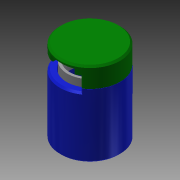
# Autodesk Inventor part: microscope_iphone_adapter
Saved by Autodesk Inventor 2014 (Build 180170000, 170)
## iProperties
Created: 2015-01-25
Part Number: microscope_iphone_adapter
Material: Generic
Document SubType Name: Modeling
Designer: caleb
Density: 1 g/cm^3
Appearance: Default
Author: caleb
Autodesk Inventor part; units mm, degrees
ref_plane "YZ Plane" through (0, 0, 0) normal (1, 0, 0) x (0, 1, 0)
ref_plane "XZ Plane" through (0, 0, 0) normal (0, 1, 0) x (-1, 0, 0)
ref_plane "XY Plane" through (0, 0, 0) normal (0, 0, 1) x (1, 0, 0)
sketch "Sketch1" plane through (0, 0, 0) normal (0, 0, 1) x (1, 0, 0)
  circle A0 centre (0, 0) radius 13.5
  dimension "d0" = 27
  constraints: 1 centre point, 1 coincident
  measures "d0" diameter of A0
extrude "Extrusion1" add sketch "Sketch1" against normal blind 25
ref_plane "Work Plane1" through (0, 0, 11) normal (0, 0, 1) x (1, 0, 0)
sketch "Sketch2" plane through (0, 0, 11) normal (0, 0, 1) x (1, 0, 0)
  circle A0 centre (0, 0) radius 13.9
  circle A1 centre (0, 0) radius 17.9
  circle A2 centre (0, 0) radius 13.5 construction
  dimension "d4" = 0.4
  dimension "d5" = 4
  constraints: 2 centre point, 2 coincident
  measures "d4" radial gap between concentric circles of A0 A2
  measures "d5" radial gap between concentric circles of A0 A1
extrude "Extrusion2" add sketch "Sketch2" against normal blind 36 separate body
sketch "Sketch3" plane through (0, 0, 11) normal (0, 0, 1) x (1, 0, 0)
  line L0 (9.28, 7.35) -> (-49.29, 7.35)
  line L1 (-49.29, 7.35) -> (-49.29, -116.48)
  line L2 (-49.29, -116.48) -> (9.28, -116.48)
  line L3 (9.28, -116.48) -> (9.28, 7.35)
  point P0 (0, 0)
  dimension "d8" = 58.57
  dimension "d9" = 123.83
  dimension "d10" = 9.28
  dimension "d11" = 7.35
  constraints: 8 end point, 2 parallel, 1 horizontal, 1 perpendicular
  measures "d8" distance of L1.end L2.end
  measures "d9" distance of L0.end L1.end
  measures "d10" distance from line of L3 point (0, 0)
  measures "d11" distance from line of L0 point (0, 0)
extrude "Extrusion3" add sketch "Sketch3" along normal blind 8.1 separate body
sketch "Sketch6" plane through (-49.29, 7.35, 11) normal (0, 1, 0) x (1, 0, 0)
  line L0 (58.57, 0) -> (0, 0) projected
  line L1 (0, 0) -> (0, -8.1) projected
  line L2 (58.57, -8.1) -> (0, -8.1) projected
  line L3 (58.57, 0) -> (58.57, -8.1) projected
  line L4 (38.77, -2.7) -> (49.27, -2.7)
  line L5 (49.27, -2.7) -> (49.27, -5.4)
  line L6 (49.27, -5.4) -> (38.77, -5.4)
  line L7 (38.77, -5.4) -> (38.77, -2.7)
  point P0 (49.29, 11)
  point P1 (49.27, -4.05)
  point P2 (58.57, -4.05)
  dimension "d20" = 10.5
  dimension "d21" = 2.7
  dimension "d22" = 9.3
  constraints: 8 end point, 2 midpoint, 2 parallel, 1 horizontal, 1 horizontal alignment, 1 perpendicular
  measures "d20" distance of L5.end L6.end
  measures "d21" distance of L4.end L5.end
  measures "d22" distance between parallel lines of L3 L5
extrude "Extrusion6" add sketch "Sketch6" along normal blind 1.08 contours L4 L5 L6 L7 bodies 3
fillet "Fillet1" radius 6 4 edges at (9.28, 7.35, 15.05) (-49.29, 7.35, 15.05) (9.28, -116.48, 15.05) (-49.29, -116.48, 15.05)
ref_plane "Work Plane2" through (0, 0, 20.9) normal (0, 0, 1) x (1, 0, 0)
sketch "Sketch4" plane through (0, 0, 11) normal (0, 0, 1) x (1, 0, 0)
  circle A0 centre (0, 0) radius 13.9 projected
  circle A1 centre (0, 0) radius 17.9 projected
extrude "Extrusion4" add sketch "Sketch4" along normal up to surface (9.9 mm away) bodies 2
sketch "Sketch5" plane through (0, 0, 20.9) normal (0, 0, 1) x (1, 0, 0)
  circle A0 centre (0, 0) radius 17.9 projected
extrude "Extrusion5" add sketch "Sketch5" along normal blind 4 bodies 2
combine bodies "Combine1" operation type subtract main body 2 bodies to subtract 3 keep tools yes
sketch "Sketch7" plane through (0, 0, 19.1) normal (0, 0, 1) x (1, 0, 0)
  arc A0 (-49.29, -110.48) -> (-43.29, -116.48) centre (-43.29, -110.48) ccw construction
  line L0 (-49.29, 1.35) -> (-49.29, -110.48) construction
  arc A1 (-43.29, 7.35) -> (-49.29, 1.35) centre (-43.29, 1.35) ccw construction
  line L1 (3.28, 7.35) -> (-43.29, 7.35) projected
  arc A2 (9.28, 1.35) -> (3.28, 7.35) centre (3.28, 1.35) ccw projected
  line L2 (9.28, -110.48) -> (9.28, 1.35) projected
  arc A3 (3.28, -116.48) -> (9.28, -110.48) centre (3.28, -110.48) ccw construction
  line L3 (-43.29, -116.48) -> (3.28, -116.48) construction
  line L4 (-0.02, 7.35) -> (-10.52, 7.35) construction
  line L5 (-0.02, 7.35) -> (-10.52, 7.35) construction
  line L6 (-0.02, 7.35) -> (-0.02, 8.43) construction
  line L7 (-10.52, 8.43) -> (-0.02, 8.43) construction
  line L8 (-10.52, 7.35) -> (-10.52, 8.43) construction
  circle A4 centre (0, 0) radius 13.9 construction
  circle A5 centre (0, 0) radius 17.9 construction
  arc A6 (9.28, -10.3485) -> (0.48, 13.8917) centre (0, 0) ccw
  line L9 (0.48, 13.8917) -> (0.48, 7.35)
  dimension "d25" = 0.5
  constraints: 4 point on circle, 2 concentric, 2 end point, 2 point on line, 1 centre point, 1 vertical
  measures "d25" distance between parallel lines of L9 L6
extrude "Extrusion7" add sketch "Sketch7" against normal blind 4 bodies 2
extrude "Extrusion8" add sketch "Sketch7" along normal up to next bodies 2
sketch "Sketch8" plane through (0, 0, 20.9) normal (0, 0, -1) x (-1, 0, 0)
  line L0 (-0.48, 13.8917) -> (-0.48, 7.35) projected
  line L1 (-0.48, 7.35) -> (-3.28, 7.35) projected
  arc A0 (-3.28, 7.35) -> (-9.28, 1.35) centre (-3.28, 1.35) ccw projected
  line L2 (-9.28, 1.35) -> (-9.28, -10.3485) projected
  arc A1 (-9.28, -10.3485) -> (-0.48, 13.8917) centre (0, 0) ccw projected
sketch "Sketch9" plane through (0, 0, 0) normal (1, 0, 0) x (0, 1, 0)
  line L0 (13.8917, 20.9) -> (7.35, 20.9) construction
  line L1 (7.35, 20.9) -> (1.35, 20.9) construction
  line L2 (1.35, 20.9) -> (-10.3485, 20.9) construction
  line L3 (13.8917, 20.9) -> (-10.3485, 20.9) construction
  line L4 (17.9, 24.9) -> (-17.9, 24.9) construction
  line L5 (-17.9, 24.9) -> (-17.9, 22.1)
  line L6 (-17.9, 22.1) -> (4.1, 20.9)
  line L7 (10.6209, 24.9) -> (-17.9, 24.9) construction
  line L8 (-10.3485, 19.1) -> (7.35, 19.1) construction
  line L9 (-15.3066, 19.1) -> (-10.3485, 19.1) construction
  line L10 (7.35, 19.1) -> (-15.3066, 19.1) construction
  line L11 (-17.9, 22.1) -> (-17.9, 19.1)
  line L12 (-17.9, 19.1) -> (4.1, 19.1)
  line L13 (4.1, 19.1) -> (4.1, 20.9)
  point P0 (0, 0)
  dimension "d30" = 22
  dimension "d31" = 3
  constraints: 12 end point, 3 point on line, 2 perpendicular, 1 collinear, 1 horizontal, 1 vertical
  measures "d30" horizontal distance of L5.end L6.end
  measures "d31" vertical distance of L5.end L9.start
extrude "Extrusion9" cut sketch "Sketch9" along normal mid plane 13 bodies 2
ref_plane "Work Plane3" through (-14.0596, 7.35, 19.1) normal (0, 0, -1) x (-1, 0, 0)
ref_plane "Work Plane4" through (-16.3214, 7.35, 11) normal (0, 0, 1) x (1, 0, 0)
split body "Split2" result two bodies by plane through (-16.3214, 7.35, 11) normal (0, 0, 1) bodies 2 first body at (-14.3004, 9.9125, 18.3333)
sketch "Sketch11" plane through (-11.7978, 7.35, 11) normal (0, 0, -1) x (-1, 0, 0)
  arc A0 (4.5236, 0) -> (-21.0778, -22.6566) centre (-11.7978, -7.35) ccw projected
  line L0 (4.5236, 0) -> (0, 0) projected
  arc A1 (0, 0) -> (-21.0778, -17.6985) centre (-11.7978, -7.35) ccw projected
  line L1 (-21.0778, -17.6985) -> (-21.0778, -22.6566) projected
  arc A2 (2.863, 0) -> (-21.0778, -20.8719) centre (-11.7978, -7.35) ccw
  arc A3 (4.5236, 0) -> (-21.0778, -22.6566) centre (-11.7978, -7.35) ccw projected
  arc A4 (2.3014, 0) -> (-21.0778, -20.2609) centre (-11.7978, -7.35) ccw
  circle A5 centre (-11.7978, -7.35) radius 17.9 projected
  circle A6 centre (-11.7978, -7.35) radius 13.9 projected
  dimension "d39" = 1.5
  dimension "d40" = 0.5
  constraints: 4 point on circle, 4 point on line, 2 centre point, 2 concentric
  measures "d39" radial gap between concentric circles of A0 A2
  measures "d40" radial gap between concentric circles of A2 A4
extrude "Extrusion10" cut sketch "Sketch11" against normal blind 2.1 contours L0 A2 L1 A0 | L0 A4 L1 A2 bodies 4
extrude "Extrusion11" add sketch "Sketch11" against normal blind 2 contours L0 A2 L1 A0 bodies 5
chamfer "Chamfer1" distance 1 angle 45 11 edges at (9.28, -15.3066, 16.1) (7.9197, -16.0527, 19.1) (6.5, -16.6781, 20.5667) (3.3069, -17.5919, 22.0832) (-3.3069, -17.5919, 22.0832) (-6.5, -16.6781, 20.5667) (-16.5693, -6.7726, 19.1) (-16.3214, 7.35, 16.1) (-16.3214, 7.35, 12) (-11.8628, -13.4046, 11) (9.28, -15.3066, 12)
chamfer "Chamfer2" distance 1 angle 45 3 edges at (-17.9, 0, 24.9) (-13.9, 0, -25) (-17.9, 0, -25)
sketch "Sketch12" plane through (-11.7978, 7.35, 13) normal (0, 0, 1) x (1, 0, 0)
  line L0 (10.2978, -7.35) -> (13.2978, -7.35)
  line L1 (13.2978, -7.35) -> (13.2978, 22.65)
  line L2 (13.2978, 22.65) -> (10.2978, 22.65)
  line L3 (10.2978, 22.65) -> (10.2978, -7.35)
  line L4 (9.8978, -7.75) -> (13.6978, -7.75)
  line L5 (13.6978, -7.75) -> (13.6978, 23.05)
  line L6 (13.6978, 23.05) -> (9.8978, 23.05)
  line L7 (9.8978, 23.05) -> (9.8978, -7.75)
  arc A0 (21.9181, -22.1145) -> (-4.0877, 0.9) centre (11.7978, -7.35) ccw construction
  circle A1 centre (11.7978, -7.35) radius 13.9 construction
  arc A2 (13.2978, 10.487) -> (10.2978, 10.487) centre (11.7978, -7.35) ccw
  arc A3 (13.2978, 6.4688) -> (10.2978, 6.4688) centre (11.7978, -7.35) ccw
  dimension "d51" = 3
  dimension "d52" = 30
  dimension "d53" = 0.4
  constraints: 16 end point, 8 point on circle, 4 parallel, 4 point on line, 2 centre point, 2 concentric, 2 perpendicular, 1 coincident, 1 horizontal, 1 midpoint, 3 other
  measures "d51" distance of L0.start L0.end
  measures "d52" distance of L0.end L1.end
  measures "d53" distance between parallel lines of L3 L7
extrude "Extrusion12" cut sketch "Sketch12" against normal up to surface (2 mm away) contours L3 A3 L1 L0 | L3 A2 L1 A3 | L3 L2 L1 A2 | L7 L6 L5 L4 bodies 5
extrude "Extrusion13" add sketch "Sketch12" against normal up to surface (2 mm away) contours L3 A2 L1 A3 bodies 4
sketch "Sketch13" plane through (0, 0, 15.1) normal (0, 0, -1) x (-1, 0, 0)
  circle A0 centre (0, 0) radius 13.9 construction
  circle A1 centre (0, 0) radius 13.9 construction
  circle A2 centre (0, 0) radius 13.5
  circle A3 centre (0, 0) radius 12
  dimension "d58" = 0.4
  dimension "d59" = 1.5
  constraints: 2 centre point
  measures "d58" radial gap between concentric circles of A0 A2
  measures "d59" radial gap between concentric circles of A2 A3
extrude "Extrusion14" add sketch "Sketch13" along normal blind 11 separate body
equation "\"d0\" = eyepiece_diameter"
equation "\"d8\" = iphone_width"
equation "\"d9\" = iphone_height"
equation "\"d10\" = iphone_camera_x"
equation "\"d11\" = iphone_camera_y"
equation "\"d20\" = iphone_sleepwake_length"
equation "\"d21\" = iphone_sleepwake_width"
equation "\"d22\" = iphone_sleepwake_offset"
equation "\"d23\" = iphone_sleepwake_height"
equation "\"d14\" = iphone_cornder_radius"
equation "\"d60\" = focus_offset"
equation "\"eyepiece_diameter\" = 27"
equation "\"focus_offset\" = 11"
equation "\"d3\" = focus_offset"
equation "\"iphone_width\" = 58.57"
equation "\"iphone_height\" = 123.83"
equation "\"iphone_thickness\" = 7.6"
equation "\"iphone_camera_x\" = 9.28"
equation "\"iphone_camera_y\" = 7.35"
equation "\"iphone_cornder_radius\" = 6"
equation "\"iphone_sleepwake_width\" = 2.7"
equation "\"iphone_sleepwake_length\" = 10.5"
equation "\"iphone_sleepwake_offset\" = 9.3"
equation "\"iphone_sleepwake_height\" = 1.08"
body "Solid1"
body "Solid3"
